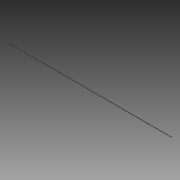
# Autodesk Inventor part: DR1-2000
Saved by Autodesk Inventor 2011 SP1 (Build 150282100, 282)
## iProperties
Created: 2018-06-30
Part Number: DR1-2000
Catalog Web Link: www.cadenas.de
Description: Molded Flexible Racks (DR)-
Vendor: KHK
Document SubType Name: Modeling
Designer: psAdmin
Manufacturer: KHK
Mass: 51.5726 g
Surface Area: 558.26 cm^2
Volume: 51.5726 cm^3
Density: 1 g/cm^3
Category: PARTsolutions
Company: KHK
Title: DR1-2000
Author: Cadenas PARTsolutions
PSOL_IDENT_0: {$CADENAS_DATA\23d-libs\khk\racks\molded_flexible_racks_dr.prj},178 {VTYP=3D},{NB=DR1-2000},{LINA=DR
PSOL_IDENT_1: 1-2000},{NN=Molded Flexible Racks (DR)},{DATE=17.03.2017 04:27:31},{GEOMDATE=27.06.2013 07:10:00},{V
PSOL_IDENT_2: ERSION=},{LINEID=30},{LINESUBID=-1},{WBVAR=}  {NB=DR1-2000},{LINA=DR1-2000},{KT=DUMMY},{CN=DR1-2000}
PSOL_IDENT_3: ,{M=1.0},{A=2000},{B=5.0},{B1=4},{C=4.3},{D=3.3},{E=2.0},{F=0.9},{G=4.9},{H=10},{ENT=632},{S=R4},{WM
PSOL_IDENT_4: F=R4001.WMF},{R=1.1}
NN: Molded Flexible Racks (DR)
NB: DR1-2000
NBSYN: $CN.
LINA: DR1-2000
CN: DR1-2000
M: 1.0
A: 2000
B: 5.0
B1: 4
C: 4.3
D: 3.3
E: 2.0
F: 0.9
G: 4.9
H: 10
ENT: 632
S: R4
SUPPLIER: KHK
ARTICLENO: DR1-2000
BOMINFO: DR1-2000
CREATOR: CADENAS GmbH
Autodesk Inventor part; units mm, degrees
ref_plane "YZ Plane" through (0, 0, 0) normal (1, 0, 0) x (0, 1, 0)
ref_plane "XZ Plane" through (0, 0, 0) normal (0, 1, 0) x (-1, 0, 0)
ref_plane "XY Plane" through (0, 0, 0) normal (0, 0, 1) x (1, 0, 0)
sketch "Sketch_1" plane through (0, 0, 0) normal (1, 0, 0) x (0, 0, -1)
  line L0 (-5, 0.9) -> (-5, 0)
  line L1 (-5, 0) -> (-2.45, 0)
  line L2 (-2.45, 0) -> (-2, 0.9)
  line L3 (-2, 0.9) -> (2, 0.9)
  line L4 (2, 0.9) -> (2.45, 0)
  line L5 (2.45, 0) -> (5, 0)
  line L6 (5, 0) -> (5, 0.9)
  arc A0 (5, 0.9) -> (3.9, 2) centre (3.9, 0.9) ccw
  line L7 (3.9, 2) -> (2.5, 2)
  line L8 (2.5, 2) -> (2, 4.3)
  line L9 (2, 4.3) -> (-2, 4.3)
  line L10 (-2, 4.3) -> (-2.5, 2)
  line L11 (-2.5, 2) -> (-3.9, 2)
  arc A1 (-3.9, 2) -> (-5, 0.9) centre (-3.9, 0.9) ccw
  constraints: 24 end point, 4 point on circle, 2 centre point
extrude "Extrusion1" add sketch "Sketch_1" along normal blind 2000
sketch "Sketch_2" plane through (0, 0, 0) normal (0, 0, 1) x (1, 0, 0)
  line L0 (-2, 8.6) -> (-2, 2)
  line L1 (-2, 2) -> (0.3589, 2)
  line L2 (0.3589, 2) -> (1.1961, 4.3)
  line L3 (1.1961, 4.3) -> (1.9471, 4.3)
  line L4 (1.9471, 4.3) -> (2.7843, 2)
  line L5 (2.7843, 2) -> (3.4989, 2)
  line L6 (3.4989, 2) -> (4.3361, 4.3)
  line L7 (4.3361, 4.3) -> (5.0887, 4.3)
  line L8 (5.0887, 4.3) -> (5.9258, 2)
  line L9 (5.9258, 2) -> (6.6389, 2)
  line L10 (6.6389, 2) -> (7.4761, 4.3)
  line L11 (7.4761, 4.3) -> (1992.5239, 4.3)
  line L12 (1992.5239, 4.3) -> (1993.3611, 2)
  line L13 (1993.3611, 2) -> (1994.0742, 2)
  line L14 (1994.0742, 2) -> (1994.9113, 4.3)
  line L15 (1994.9113, 4.3) -> (1995.6639, 4.3)
  line L16 (1995.6639, 4.3) -> (1996.5011, 2)
  line L17 (1996.5011, 2) -> (1997.2157, 2)
  line L18 (1997.2157, 2) -> (1998.0529, 4.3)
  line L19 (1998.0529, 4.3) -> (1998.8039, 4.3)
  line L20 (1998.8039, 4.3) -> (1999.6411, 2)
  line L21 (1999.6411, 2) -> (2002, 2)
  line L22 (2002, 2) -> (2002, 8.6)
  line L23 (2002, 8.6) -> (-2, 8.6)
  constraints: 48 end point
extrude "Extrusion2" cut sketch "Sketch_2" along normal mid plane 10
body "Solid1"
